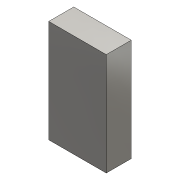
# Autodesk Inventor part: BLANK-BC-10007
Saved by Autodesk Inventor 2016 (Build 200138000, 138)
## iProperties
Created: 2015-12-02
Part Number: BLANK-BC-10007
Material: Aço Carbono
Document SubType Name: Modeling
Designer: reinaldo.basilio
Density: 7.87 g/cm^3
Appearance: Semi-Polished
Mass: 10907.8 g
Surface Area: 867 cm^2
Volume: 1386 cm^3
Project: DIPOLO BC-3T- SIRIUS
Cost Center: 1504002005
Description: Peça frontal para fechar circuito  magnético.
Author: reinaldo.basilio
Title: DIPOLO BC-3T- SIRIUS
Subject: BLANK-BC-10007
Autodesk Inventor part; units mm, degrees
ref_plane "YZ Plane" through (0, 0, 0) normal (1, 0, 0) x (0, 1, 0)
ref_plane "XZ Plane" through (0, 0, 0) normal (0, 1, 0) x (-1, 0, 0)
ref_plane "XY Plane" through (0, 0, 0) normal (0, 0, 1) x (1, 0, 0)
sketch "Sketch1" plane through (0, 0, 0) normal (0, 1, 0) x (-1, 0, 0)
  line L0 (57.5, 102.5) -> (-57.5, 102.5)
  line L1 (-57.5, 102.5) -> (-57.5, -102.5)
  line L2 (-57.5, -102.5) -> (57.5, -102.5)
  line L3 (57.5, -102.5) -> (57.5, 102.5)
  point P0 (0, 0)
  point P1 (0, -102.5)
  point P2 (-57.5, 0)
  dimension "d0" = 115
  dimension "d1" = 205
  constraints: 8 end point, 2 midpoint, 2 parallel, 1 horizontal, 1 horizontal alignment, 1 perpendicular, 1 vertical alignment
  measures "d0" distance of L1.end L2.end
  measures "d1" distance of L2.end L0.start
extrude "Extrusion1" add sketch "Sketch1" along normal blind 50
body "Solid1"
